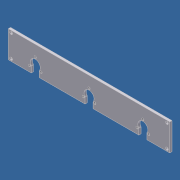
# Autodesk Inventor part: Top
Saved by Autodesk Inventor 2012 SP1 (Build 160190100, 190)
## iProperties
Created: 2010-12-14
Part Number: Top
Document SubType Name: Modeling
Designer: berny
Density: 2.71 g/cm^3
Material: Aluminum-6061
Mass: 542.356 g
Surface Area: 728.987 cm^2
Volume: 200.131 cm^3
Author: berny
Autodesk Inventor part; units mm, degrees
ref_plane "YZ Plane" through (0, 0, 0) normal (1, 0, 0) x (0, 1, 0)
ref_plane "XZ Plane" through (0, 0, 0) normal (0, 1, 0) x (-1, 0, 0)
ref_plane "XY Plane" through (0, 0, 0) normal (0, 0, 1) x (1, 0, 0)
sketch "Sketch1" plane through (0, 0, 0) normal (0, 0, 1) x (1, 0, 0)
  line L0 (0, 0) -> (457.2, 0)
  line L1 (457.2, 0) -> (457.2, 76.2)
  line L2 (457.2, 76.2) -> (0, 76.2)
  line L3 (0, 76.2) -> (0, 0)
  dimension "d0" = 76.2
  dimension "d1" = 457.2
  constraints: 8 end point, 2 parallel, 1 horizontal, 1 perpendicular
  measures "d0" distance of L2.end L0.start
  measures "d1" distance between parallel lines of L1 L3
extrude "Extrusion1" add sketch "Sketch1" along normal blind 6.35
sketch "Sketch2" plane through (0, 0, 6.35) normal (0, 0, 1) x (1, 0, 0)
  line L0 (0, 0) -> (0, 76.2) projected
  line L1 (457.2, 0) -> (0, 0) projected
  circle A0 centre (76.2, 25.4) radius 14.2875
  line L2 (64.77, 16.8275) -> (64.77, 0)
  line L3 (87.63, 16.8275) -> (87.63, 0)
  circle A1 centre (228.6, 25.4) radius 14.2875
  line L4 (217.17, 16.8275) -> (217.17, 0)
  line L5 (240.03, 16.8275) -> (240.03, 0)
  circle A2 centre (381, 25.4) radius 14.2875
  line L6 (369.57, 16.8275) -> (369.57, 0)
  line L7 (392.43, 16.8275) -> (392.43, 0)
  circle A3 centre (533.4, 25.4) radius 14.2875
  line L8 (521.97, 16.8275) -> (521.97, 0)
  line L9 (544.83, 16.8275) -> (544.83, 0)
  circle A4 centre (685.8, 25.4) radius 14.2875
  line L10 (674.37, 16.8275) -> (674.37, 0)
  line L11 (697.23, 16.8275) -> (697.23, 0)
  circle A5 centre (838.2, 25.4) radius 14.2875
  line L12 (826.77, 16.8275) -> (826.77, 0)
  line L13 (849.63, 16.8275) -> (849.63, 0)
  line L14 (217.17, 0) -> (240.03, 0)
  line L15 (369.57, 0) -> (392.43, 0)
  line L16 (521.97, 0) -> (544.83, 0)
  line L17 (671.8667, 0) -> (697.23, 0)
  line L18 (826.77, 0) -> (849.63, 0)
  line L19 (674.37, 0) -> (697.23, 0)
  dimension "d4" = 22.86
  dimension "d5" = 11.43
  dimension "d6" = 11.43
  dimension "d7" = 25.4
  dimension "d8" = 28.575
  dimension "d9" = 76.2
  dimension "d17" = 152.4
  constraints: 36 end point, 12 point on circle, 6 centre point, 6 collinear, 3 point on line, 2 perpendicular, 1 horizontal, 40 other
  measures "d4" distance between parallel lines of L3 L2
  measures "d5" distance from line of L2 A0.centre
  measures "d6" distance from line of L3 A0.centre
  measures "d7" distance from line of L1 A0.centre
  measures "d8" diameter of A0
  measures "d9" distance from line of L0 A0.centre
  measures "d17" distance of A0.centre A1.centre
extrude "Extrusion4" cut sketch "Sketch2" against normal up to next
sketch "Sketch3" plane through (0, 0, 6.35) normal (0, 0, 1) x (1, 0, 0)
  arc A0 (87.63, 16.8275) -> (64.77, 16.8275) centre (76.2, 25.4) ccw projected
  line L0 (217.17, 0) -> (87.63, 0) projected
  point P0 (76.2, 44.4)
  point P1 (59.7455, 15.9)
  point P2 (92.6545, 15.9)
  point P3 (228.6, 44.4)
  point P4 (212.1455, 15.9)
  point P5 (245.0545, 15.9)
  point P6 (381, 44.4)
  point P7 (364.5455, 15.9)
  point P8 (397.4545, 15.9)
  point P9 (533.4, 44.4)
  point P10 (516.9455, 15.9)
  point P11 (549.8545, 15.9)
  point P12 (685.8, 44.4)
  point P13 (669.3455, 15.9)
  point P14 (702.2545, 15.9)
  point P15 (838.2, 44.4)
  point P16 (821.7455, 15.9)
  point P17 (854.6545, 15.9)
  dimension "d23" = 19
  dimension "d26" = 360
  dimension "d33" = 152.4
  dimension "d53" = 120
  dimension "d54" = 120
  dimension "d55" = 19
  constraints: 1 horizontal, 19 other
  measures "d23" distance of A0.centre point (76.2, 44.4)
  measures "d33" distance of point (76.2, 44.4) point (228.6, 44.4)
  measures "d55" distance of point (59.746, 15.9) A0.centre
hole "Hole1" at (76.2, 44.4, 6.35) at (59.7455, 15.9, 6.35) at (92.6545, 15.9, 6.35) at (228.6, 44.4, 6.35) at (212.1455, 15.9, 6.35) at (245.0545, 15.9, 6.35) at (381, 44.4, 6.35) at (364.5455, 15.9, 6.35) at (397.4545, 15.9, 6.35) at (533.4, 44.4, 6.35) at (516.9455, 15.9, 6.35) at (549.8545, 15.9, 6.35) at (685.8, 44.4, 6.35) at (669.3455, 15.9, 6.35) at (702.2545, 15.9, 6.35) at (838.2, 44.4, 6.35) at (821.7455, 15.9, 6.35) at (854.6545, 15.9, 6.35) direction (0, 0, -1) diameter 6.4008 end through all thread size "5/16-18 UNC" class "2B" standard "ANSI Unified Screw Threads"
sketch "Sketch4" plane through (0, 0, 6.35) normal (0, 0, 1) x (1, 0, 0)
  line L0 (457.2, 76.2) -> (457.2, 0) projected
  line L1 (0, 76.2) -> (457.2, 76.2) projected
  line L2 (0, 0) -> (0, 76.2) projected
  line L3 (64.77, 0) -> (0, 0) projected
  point P0 (7.9375, 69.85)
  point P1 (7.9375, 6.35)
  point P2 (449.2625, 6.35)
  point P3 (449.2625, 69.85)
  dimension "d42" = 6.35
  dimension "d43" = 6.35
  dimension "d44" = 7.9375
  dimension "d45" = 7.9375
  constraints: 2 horizontal alignment, 2 vertical alignment
  measures "d42" distance from line of L3 point (7.937, 6.35)
  measures "d43" distance from line of L1 point (7.937, 69.85)
  measures "d44" distance from line of L0 point (449.262, 69.85)
  measures "d45" distance from line of L2 point (7.937, 69.85)
hole "Hole2" at (7.9375, 69.85, 6.35) at (7.9375, 6.35, 6.35) at (449.2625, 6.35, 6.35) at (449.2625, 69.85, 6.35) direction (0, 0, -1) diameter 4.4958 end through all counterbore diameter 7.9502 counterbore depth 4.1656 clearance for "Socket Head Cap Screw" size "#8" standard "Ansi Unified Screw Threads"
sketch "Sketch5" plane through (0, 0, 6.35) normal (0, 0, 1) x (1, 0, 0)
  circle A0 centre (449.2625, 69.85) radius 3.9751 projected
  circle A1 centre (449.2625, 6.35) radius 3.9751 projected
  circle A2 centre (7.9375, 6.35) radius 3.9751 projected
  circle A3 centre (7.9375, 69.85) radius 3.9751 projected
  circle A4 centre (397.4545, 15.9) radius 3.2004 projected
  circle A5 centre (364.5455, 15.9) radius 3.2004 projected
  circle A6 centre (381, 44.4) radius 3.2004 projected
  circle A7 centre (245.0545, 15.9) radius 3.2004 projected
  circle A8 centre (212.1455, 15.9) radius 3.2004 projected
  circle A9 centre (228.6, 44.4) radius 3.2004 projected
  circle A10 centre (92.6545, 15.9) radius 3.2004 projected
  circle A11 centre (59.7455, 15.9) radius 3.2004 projected
  circle A12 centre (76.2, 44.4) radius 3.2004 projected
  line L0 (369.57, 0) -> (369.57, 16.8275) projected
  arc A13 (392.43, 16.8275) -> (369.57, 16.8275) centre (381, 25.4) ccw projected
  line L1 (392.43, 16.8275) -> (392.43, 0) projected
  line L2 (457.2, 0) -> (392.43, 0) projected
  line L3 (457.2, 76.2) -> (457.2, 0) projected
  line L4 (0, 76.2) -> (457.2, 76.2) projected
  line L5 (0, 0) -> (0, 76.2) projected
  line L6 (64.77, 0) -> (0, 0) projected
  line L7 (64.77, 0) -> (64.77, 16.8275) projected
  arc A14 (87.63, 16.8275) -> (64.77, 16.8275) centre (76.2, 25.4) ccw projected
  line L8 (87.63, 16.8275) -> (87.63, 0) projected
  line L9 (217.17, 0) -> (87.63, 0) projected
  line L10 (217.17, 0) -> (217.17, 16.8275) projected
  arc A15 (240.03, 16.8275) -> (217.17, 16.8275) centre (228.6, 25.4) ccw projected
  line L11 (240.03, 16.8275) -> (240.03, 0) projected
  line L12 (369.57, 0) -> (240.03, 0) projected
  circle A16 centre (92.6545, 15.9) radius 3.9688
  line L13 (88.6857, 18.4546) -> (89.3174, 18.0482)
  dimension "d56" = 7.9375
  dimension "d57" = 0.7511
  constraints: 2 end point, 1 coincident, 1 point on circle, 3 other
  measures "d57" distance of L13.start L13.end
body "Solid1"
